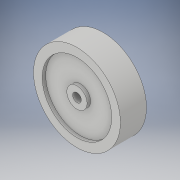
# Autodesk Inventor part: SubWheelWithHole
Saved by Autodesk Inventor 2017 (Build 210142000, 142)
## iProperties
Created: 2016-09-24
Part Number: SubWheelWithHole
Material: Generic
Document SubType Name: Modeling
Designer: vslabsal
Density: 1 g/cm^3
Appearance: Default
Author: vslabsal
Autodesk Inventor part; units mm, degrees
ref_plane "YZ Plane" through (0, 0, 0) normal (1, 0, 0) x (0, 1, 0)
ref_plane "XZ Plane" through (0, 0, 0) normal (0, 1, 0) x (-1, 0, 0)
ref_plane "XY Plane" through (0, 0, 0) normal (0, 0, 1) x (1, 0, 0)
sketch "Sketch3" plane through (0, 0, 0) normal (0, 0, 1) x (1, 0, 0)
  circle A0 centre (0, 0) radius 63.5
  dimension "d1" = 127
  constraints: 1 centre point, 1 coincident
  measures "d1" diameter of A0
extrude "Extrusion1" add sketch "Sketch3" along normal blind 38.1
sketch "Sketch4" plane through (0, 0, 38.1) normal (0, 0, 1) x (1, 0, 0)
  circle A0 centre (0, 0) radius 6.35
  dimension "d4" = 12.7
  constraints: 1 centre point, 1 coincident
  measures "d4" diameter of A0
hole "Hole1" at (0, 0, 38.1) direction (0, 0, -1) diameter 12.7 end through all
sketch "Sketch5" plane through (0, 0, 38.1) normal (0, 0, 1) x (1, 0, 0)
  circle A0 centre (0, 0) radius 50.8
  circle A1 centre (0, 0) radius 14.861
  dimension "d12" = 101.6
  dimension "d13" = 29.722
  constraints: 2 centre point, 2 coincident
  measures "d12" diameter of A0
  measures "d13" diameter of A1
emboss "Emboss1" sketch "Sketch5" operation cut depth 5.08 direction (0, 0, -1)
sketch "Sketch6" plane through (0, 0, 0) normal (0, 0, -1) x (-1, 0, 0)
  circle A0 centre (0, 0) radius 50.8
  circle A1 centre (0, 0) radius 14.861
  dimension "d16" = 101.6
  dimension "d17" = 29.722
  constraints: 2 centre point, 2 coincident
  measures "d16" diameter of A0
  measures "d17" diameter of A1
emboss "Emboss2" sketch "Sketch6" operation cut depth 5.08 direction (0, 0, 1)
body "Solid1"
